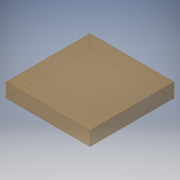
# Autodesk Inventor part: Tile
Saved by Autodesk Inventor 2016 (Build 200138000, 138)
## iProperties
Created: 2015-08-29
Part Number: Tile
Material: Polycarbonate, Smoke
Document SubType Name: Modeling
Designer: Pranav
Density: 1.2 g/cm^3
Appearance: Polycarbonate - Smoked
Author: Pranav
Autodesk Inventor part; units mm, degrees
ref_plane "YZ Plane" through (0, 0, 0) normal (1, 0, 0) x (0, 1, 0)
ref_plane "XZ Plane" through (0, 0, 0) normal (0, 1, 0) x (-1, 0, 0)
ref_plane "XY Plane" through (0, 0, 0) normal (0, 0, 1) x (1, 0, 0)
sketch "Sketch1" plane through (0, 0, 0) normal (0, 1, 0) x (-1, 0, 0)
  line L0 (0, 0) -> (304.8, 0)
  line L1 (304.8, 0) -> (304.8, -304.8)
  line L2 (304.8, -304.8) -> (0, -304.8)
  line L3 (0, -304.8) -> (0, 0)
  dimension "d0" = 304.8
  dimension "d1" = 304.8
  constraints: 8 end point, 2 parallel, 1 horizontal, 1 perpendicular
  measures "d0" distance of L1.end L2.end
  measures "d1" distance of L0.end L1.end
extrude "Extrusion1" add sketch "Sketch1" along normal blind 50.8
body "Solid1"
